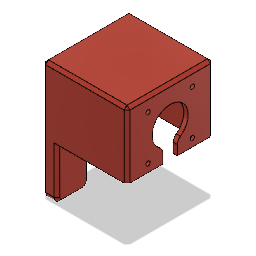
Motor-mounting-blockV2 v12 (Autodesk Fusion 360 design; units mm, degrees)
Autodesk Fusion 360 part; units mm, degrees
sketch "Sketch1" plane through (0, 0, 0) normal (1, 0, 0) x (0, 0, -1)
  line L0 (35, -21.15) -> (-35, -21.15)
  line L1 (-15.5, 15.5) -> (15.5, 15.5) construction
  line L2 (15.5, 15.5) -> (15.5, -15.5) construction
  line L3 (15.5, -15.5) -> (-15.5, -15.5) construction
  line L4 (-15.5, -15.5) -> (-15.5, 15.5) construction
  circle A0 centre (-15.5, 15.5) radius 1.5
  circle A1 centre (15.5, 15.5) radius 1.5
  circle A2 centre (15.5, -15.5) radius 1.5
  circle A3 centre (-15.5, -15.5) radius 1.5
  circle A4 centre (0, 0) radius 12.5
  line L5 (21.15, -21.15) -> (-21.15, -21.15)
  line L6 (-21.15, -21.15) -> (-21.15, 21.15)
  line L7 (-21.15, 21.15) -> (21.15, 21.15)
  line L8 (21.15, 21.15) -> (21.15, -21.15)
  line L9 (-35, -21.15) -> (-21.15, -21.15)
  line L10 (35, -21.15) -> (21.15, -21.15)
  line L11 (30.15, 21.15) -> (-30.15, 21.15)
  line L12 (-30.15, 21.15) -> (-30.15, -21.15)
  line L13 (-30.15, -21.15) -> (30.15, -21.15)
  line L14 (30.15, -21.15) -> (30.15, 21.15)
  line L15 (30.15, 21.15) -> (-30.15, 21.15)
  line L16 (-30.15, 21.15) -> (-30.15, 25.15)
  line L17 (-30.15, 25.15) -> (30.15, 25.15)
  line L18 (30.15, 25.15) -> (30.15, 21.15)
  line L19 (5, -21.15) -> (-5, -21.15)
  line L20 (-5, -21.15) -> (-5, 0)
  line L21 (-5, 0) -> (5, 0)
  line L22 (5, 0) -> (5, -21.15)
  line L23 (22.15, -21.15) -> (22.15, 25.15)
  line L24 (-22.15, 25.15) -> (-22.15, -21.15)
  line L25 (30.15, 22.15) -> (-30.15, 22.15)
  dimension "d3" = 3
  dimension "d4" = 3
  dimension "d5" = 3
  dimension "d6" = 3
  dimension "d7" = 31
  dimension "d8" = 31
  dimension "d11" = 25
  dimension "d12" = 42.3
  dimension "d13" = 42.3
  dimension "d45" = 21.15
  dimension "d46" = 15.5
  dimension "d69" = 21.15
  dimension "d110" = 10
  dimension "d111" = 5
  dimension "d123" = 1
  dimension "d124" = 1
  dimension "d125" = 1
  dimension "d129" = 15.5
  dimension "d130" = 8
  dimension "d131" = 8
  dimension "d136" = 3
  measures "d3" diameter of A0
  measures "d4" diameter of A1
  measures "d5" diameter of A2
  measures "d6" diameter of A3
  measures "d11" diameter of A4
  measures "d46" distance of L3
  measures "d111" distance of A4.centre
  measures "d123" distance of L8 L23
  measures "d124" distance of L6 L24
  measures "d125" distance of L15 L25
  measures "d129" distance of A4.centre
extrude "Extrude16" add sketch "Sketch1" along normal blind 3 contours L0 L10 L11 L13 L14 L15 L23 | L0 L8 L10 L11 L13 L15 L23 | L11 L15 L18 L23 L25 | L0 A4 L5 L6 L7 L8 L11 L13 L15 L20 L22 | L7 L11 L15 L23 L24 L25 | L17 L18 L23 L25 | L17 L23 L24 L25 | L0 L6 L9 L11 L13 L15 L24 | L16 L17 L24 L25 | L11 L15 L16 L24 L25 | L0 L9 L11 L12 L13 L15 L24
extrude "Extrude17" add sketch "Sketch1" against normal blind 43 contours L0 L10 L11 L13 L14 L15 L23 | L11 L15 L18 L23 L25 | L17 L18 L23 L25 | L17 L23 L24 L25 | L16 L17 L24 L25 | L11 L15 L16 L24 L25 | L0 L9 L11 L12 L13 L15 L24
sketch "Sketch15" plane through (0, -21.15, 0) normal (0, -1, 0) x (1, 0, 0)
  line L0 (0, 22.15) -> (0, 5)
  line L1 (0, 5) -> (3, 5)
  line L2 (3, 5) -> (3, 30.15)
  line L3 (3, 30.15) -> (-43, 30.15)
  line L4 (-43, 30.15) -> (-43, 22.15)
  line L5 (-43, 22.15) -> (0, 22.15)
  circle A0 centre (-2.6, 26.25) radius 2.6
  circle A1 centre (-40.4, 26.25) radius 2.6
  circle A2 centre (-40.4, -26.25) radius 2.6
  circle A3 centre (-2.6, -26.25) radius 2.6
  line L6 (-40.4, 26.25) -> (-2.6, 26.25) construction
  line L7 (-2.6, 26.25) -> (-2.6, -26.25) construction
  line L8 (-2.6, -26.25) -> (-40.4, -26.25) construction
  line L9 (-40.4, -26.25) -> (-40.4, 26.25) construction
  dimension "d139" = 5.2
  dimension "d143" = 37.8
  dimension "d144" = 52.5
  dimension "d145" = 26.25
  dimension "d151" = 2.6
  measures "d139" diameter of A1
  measures "d143" distance of origin
  measures "d145" distance of origin
  measures "d151" distance of origin
sketch "Sketch16" plane through (-43, 0, 0) normal (-1, 0, 0) x (0, 0, 1)
  line L0 (-30.15, 25.15) -> (-30.15, -21.15)
  line L1 (-30.15, -21.15) -> (-22.15, -21.15)
  line L2 (-22.15, -21.15) -> (-22.15, 22.15)
  line L3 (-22.15, 22.15) -> (22.15, 22.15)
  line L4 (22.15, 22.15) -> (22.15, -21.15)
  line L5 (22.15, -21.15) -> (30.15, -21.15)
  line L6 (30.15, -21.15) -> (30.15, 25.15)
  line L7 (30.15, 25.15) -> (-30.15, 25.15)
  line L8 (-30.15, 25.15) -> (30.15, 25.15)
  line L9 (30.15, 25.15) -> (30.15, -21.15)
  line L10 (30.15, -21.15) -> (-30.15, -21.15)
  line L11 (-30.15, -21.15) -> (-30.15, 25.15)
extrude "Extrude18" add sketch "Sketch16" along normal blind 3
extrude "Extrude19" cut sketch "Sketch15" against normal blind 7 contours A1 | A0 | A2 | A3
sketch "Sketch17" plane through (0, -14.15, 0) normal (0, -1, 0) x (1, 0, 0)
  circle A0 centre (-40.4, 26.25) radius 2.6
  circle A1 centre (-40.4, 26.25) radius 2.5
  circle A2 centre (-2.6, 26.25) radius 2.5
  circle A3 centre (-40.4, -26.25) radius 2.5
  circle A4 centre (-2.6, -26.25) radius 2.5
  circle A5 centre (-40.4, 26.25) radius 2
  circle A6 centre (-2.6, 26.25) radius 2
  circle A7 centre (-40.4, -26.25) radius 2
  circle A8 centre (-2.6, -26.25) radius 2
  line L0 (-40.4, 26.25) -> (-2.6, 26.25) construction
  line L1 (-2.6, 26.25) -> (-2.6, -26.25) construction
  line L2 (-2.6, -26.25) -> (-40.4, -26.25) construction
  line L3 (-40.4, -26.25) -> (-40.4, 26.25) construction
  dimension "d152" = 4
  dimension "d153" = 4
  dimension "d154" = 4
  dimension "d155" = 4
  dimension "d159" = 2.6
  measures "d152" diameter of A7
  measures "d153" diameter of A8
  measures "d154" diameter of A6
  measures "d155" diameter of A5
  measures "d159" distance of origin L1
extrude "Extrude20" cut sketch "Sketch17" against normal blind 10 contours A5 | A6 | A7 | A8
extrude "Extrude21" add 1 faces at (-46, 9.7167, -7.3833) along direction (-1, 0, 0) blind 10
sketch "Sketch18" plane through (0, -21.15, 0) normal (0, -1, 0) x (1, 0, 0)
  circle A0 centre (-2.6, 26.25) radius 2.6
  circle A1 centre (-2.6, -26.25) radius 2.6
  circle A2 centre (-40.4, 26.25) radius 2.6
  circle A3 centre (-40.4, -26.25) radius 2.6
  line L0 (0, 22.15) -> (0, 5)
  line L1 (0, 5) -> (3, 5)
  line L2 (3, 5) -> (3, 30.15)
  line L3 (3, 30.15) -> (-56, 30.15)
  line L4 (-56, 30.15) -> (-56, -30.15)
  line L5 (-56, -30.15) -> (3, -30.15)
  line L6 (3, -30.15) -> (3, -5)
  line L7 (3, -5) -> (0, -5)
  line L8 (0, -5) -> (0, -22.15)
  line L9 (0, -22.15) -> (-43, -22.15)
  line L10 (-43, -22.15) -> (-43, 22.15)
  line L11 (-43, 22.15) -> (0, 22.15)
  line L12 (-56, 30.15) -> (-46, 30.15)
  line L13 (-46, 30.15) -> (-46, -30.15)
  line L14 (-46, -30.15) -> (-56, -30.15)
  line L15 (-56, -30.15) -> (-56, 30.15)
  dimension "d162" = 10
  measures "d162" distance of origin
extrude "Extrude22" add sketch "Sketch18" along normal blind 37 contours L3 L4 L5 L12 L13 L14 L15
sketch "Sketch19" plane through (-56, 0, 0) normal (-1, 0, 0) x (0, 0, 1)
  line L0 (30.15, -58.15) -> (30.15, 25.15)
  line L1 (30.15, 25.15) -> (-30.15, 25.15)
  line L2 (-30.15, 25.15) -> (-30.15, -58.15)
  line L3 (-30.15, -58.15) -> (30.15, -58.15)
  line L4 (-7.5, -58.15) -> (7.5, -58.15)
  line L5 (7.5, -53.15) -> (7.5, -38.15)
  line L6 (2.5, -33.15) -> (-2.5, -33.15)
  line L7 (-7.5, -38.15) -> (-7.5, -53.15)
  arc A0 (-2.5, -33.15) -> (-7.5, -38.15) centre (-2.5, -38.15) ccw
  arc A1 (7.5, -38.15) -> (2.5, -33.15) centre (2.5, -38.15) ccw
  line L8 (-26.15, -58.15) -> (-12.5, -58.15)
  line L9 (12.5, -58.15) -> (26.15, -58.15)
  arc A2 (-12.5, -58.15) -> (-7.5, -53.15) centre (-12.5, -53.15) ccw
  arc A3 (7.5, -53.15) -> (12.5, -58.15) centre (12.5, -53.15) ccw
  line L10 (-30.15, 25.15) -> (-30.15, -54.15)
  line L11 (30.15, -54.15) -> (30.15, 25.15)
  line L12 (-30.15, 25.15) -> (30.15, 25.15)
  arc A4 (-30.15, -54.15) -> (-26.15, -58.15) centre (-26.15, -54.15) ccw
  arc A5 (26.15, -58.15) -> (30.15, -54.15) centre (26.15, -54.15) ccw
  dimension "d165" = 25
  dimension "d166" = 15
  dimension "d167" = 7.5
  dimension "d168" = 5
  dimension "d169" = 5
  dimension "d170" = 5
  dimension "d171" = 4
  measures "d167" distance of origin L5
  measures "d168" radius of A0
  measures "d169" radius of A2
  measures "d170" radius of A3
  measures "d171" radius of A4
extrude "Extrude23" cut sketch "Sketch19" against normal up to surface (10 mm away) contours L0 L3 A5 | L3 L4 L5 L6 L7 A0 A1 A2 A3 | L2 L3 A4
chamfer "Chamfer1" distance 2 angle 45 32 edges at (-26.5, 25.15, -30.15) (-56, 25.15, 0) (-26.5, 25.15, 30.15) (3, 25.15, 0) (3, 2, 30.15) (-56, -14.5, 30.15) (-56, -56.9784, 28.9784) (-56, -58.15, 19.325) (-56, -56.6855, 8.9645) (-56, -45.65, 7.5) (-56, -34.6145, 6.0355) (-56, -33.15, 0) (-56, -34.6145, -6.0355) (-56, -45.65, -7.5) (-56, -56.6855, -8.9645) (-56, -58.15, -19.325) (-56, -56.9784, -28.9784) (-56, -14.5, -30.15) (3, 2, -30.15) (-46, -37.65, 30.15) (-46, -56.9784, 28.9784) (-46, -58.15, 19.325) (-46, -56.6855, 8.9645) (-46, -45.65, 7.5) (-46, -34.6145, 6.0355) (-46, -33.15, 0) (-46, -34.6145, -6.0355) (-46, -45.65, -7.5) (-46, -56.6855, -8.9645) (-46, -58.15, -19.325) (-46, -56.9784, -28.9784) (-46, -37.65, -30.15)
fillet "Fillet12" radius 5 2 edges at (1.5, -11.4564, 5) (1.5, -11.4564, -5)
equation "d145 = ( 52.5 / 2 ) * 1 mm"
